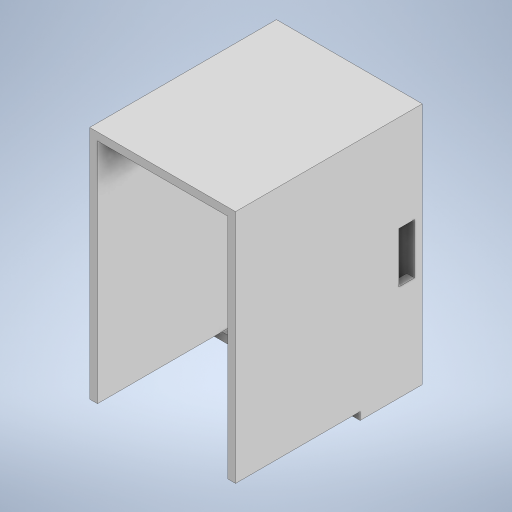
# Autodesk Inventor part: Motor_Base_3
Saved by Autodesk Inventor 2023.5 (Build 275446020, 446B)
## iProperties
Created: 2025-04-14
Part Number: Motor_Base_3
Material: Generic
Document SubType Name: Modeling
Designer: Lucky Sah
Density: 1 g/cm^3
Appearance: Default
Author: Lucky Sah
Autodesk Inventor part; units mm, degrees
ref_plane "YZ Plane" through (0, 0, 0) normal (1, 0, 0) x (0, 1, 0)
ref_plane "XZ Plane" through (0, 0, 0) normal (0, 1, 0) x (-1, 0, 0)
ref_plane "XY Plane" through (0, 0, 0) normal (0, 0, 1) x (1, 0, 0)
sketch "Sketch1" plane through (0, 0, 0) normal (0, 0, 1) x (1, 0, 0)
  line L0 (0, 0) -> (33.49, 0)
  line L1 (33.49, 0) -> (33.49, 58.49)
  line L2 (33.49, 58.49) -> (0, 58.49)
  line L3 (0, 58.49) -> (0, 0)
  line L4 (-2, 60.49) -> (35.49, 60.49)
  line L5 (35.49, 60.49) -> (35.49, -2)
  line L6 (35.49, -2) -> (-2, -2)
  line L7 (-2, -2) -> (-2, 60.49)
  dimension "d0" = 33.49
  dimension "d1" = 58.49
  dimension "d2" = 2
  constraints: 16 end point, 4 parallel, 2 perpendicular, 1 horizontal, 3 other
  measures "d0" distance of L2.end L1.end
  measures "d1" distance of L1.end L0.end
  measures "d2" distance between parallel lines of L2 L4
extrude "Extrusion1" add sketch "Sketch1" along normal blind 46
sketch "Sketch2" plane through (0, 0, 46) normal (0, 0, 1) x (1, 0, 0)
  line L0 (-2, 60.49) -> (-2, -2) projected
  line L1 (-2, 0) -> (35.49, 0)
  line L2 (35.49, -2) -> (35.49, 60.49) projected
  line L3 (-2, -2) -> (35.49, -2) projected
  line L4 (35.49, -2) -> (-2, -2)
  line L5 (-2, -2) -> (-2, 0)
  point P0 (0, 0)
  constraints: 6 end point, 2 horizontal, 2 point on line, 1 perpendicular
extrude "Extrusion2" cut sketch "Sketch2" against normal blind 32
sketch "Sketch3" plane through (0, 0, 0) normal (0, 0, -1) x (-1, 0, 0)
  line L0 (-35.49, 60.49) -> (2, 60.49) projected
  line L1 (2, -2) -> (-35.49, -2) projected
  line L2 (-35.49, 60.49) -> (2, 60.49)
  line L3 (2, 60.49) -> (2, -2)
  line L4 (2, -2) -> (-35.49, -2)
  line L5 (-35.49, -2) -> (-35.49, 60.49)
  point P0 (0, 0)
  constraints: 8 end point, 2 parallel, 1 horizontal, 1 perpendicular
extrude "Extrusion3" add sketch "Sketch3" along normal blind 2
sketch "Sketch4" plane through (-2, 0, 46) normal (-1, 0, 0) x (0, 0, 1)
  line L0 (-48, -2) -> (-48, 60.49) projected
  line L1 (-48, 35.745) -> (-42, 35.745)
  line L2 (-42, 35.745) -> (-42, 22.745)
  line L3 (-42, 22.745) -> (-48, 22.745)
  line L4 (-48, 60.49) -> (0, 60.49) projected
  line L5 (-46, 35.745) -> (-46, 22.745)
  point P0 (-46, 0)
  point P1 (-45, 22.745)
  point P2 (-45, 35.745)
  dimension "d10" = 6
  dimension "d11" = 13
  dimension "d12" = 24.745
  dimension "d13" = 2
  constraints: 8 end point, 4 point on line, 3 perpendicular, 2 midpoint, 1 horizontal
  measures "d10" distance between parallel lines of L0 L2
  measures "d11" distance of point (-45, 22.745) point (-45, 35.745)
  measures "d12" distance between parallel lines of L4 L1
  measures "d13" distance between parallel lines of L0 L5
extrude "Extrusion4" cut sketch "Sketch4" against normal up to surface (37.49 mm away) contours L5 L1 L2 L3
body "Solid1"
